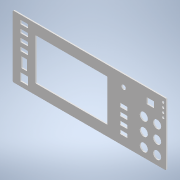
# Autodesk Inventor part: FrontPlate
Saved by Autodesk Inventor 2020.3 (Build 243373000, 373)
## iProperties
Created: 2021-02-28
Part Number: FrontPlate
Material: Generic
Document SubType Name: Modeling
Designer: vmiguel
Density: 1 g/cm^3
Appearance: Default
Author: vmiguel
Autodesk Inventor part; units mm, degrees
ref_plane "YZ Plane" through (0, 0, 0) normal (1, 0, 0) x (0, 1, 0)
ref_plane "XZ Plane" through (0, 0, 0) normal (0, 1, 0) x (-1, 0, 0)
ref_plane "XY Plane" through (0, 0, 0) normal (0, 0, 1) x (1, 0, 0)
sketch "Sketch1" plane through (0, 0, 0) normal (0, 0, 1) x (1, 0, 0)
  line L0 (-103.5, 42) -> (103.5, 42)
  line L1 (103.5, 42) -> (103.5, -42)
  line L2 (103.5, -42) -> (-103.5, -42)
  line L3 (-103.5, -42) -> (-103.5, 42)
  line L4 (-103.5, 42) -> (103.5, -42) construction
  line L5 (103.5, 42) -> (-103.5, -42) construction
  line L6 (-72.9, 28.2) -> (24.32, 28.2)
  line L7 (24.32, 28.2) -> (24.32, -28.2)
  line L8 (24.32, -28.2) -> (-72.9, -28.2)
  line L9 (-72.9, -28.2) -> (-72.9, 28.2)
  line L10 (-72.9, 28.2) -> (24.32, -28.2) construction
  line L11 (24.32, 28.2) -> (-72.9, -28.2) construction
  line L12 (-93.5, -25.4) -> (-82.9, -25.4)
  line L13 (-82.9, -25.4) -> (-82.9, -36)
  line L14 (-82.9, -36) -> (-93.5, -36)
  line L15 (-93.5, -36) -> (-93.5, -25.4)
  line L16 (-93.5, -25.4) -> (-82.9, -36) construction
  line L17 (-82.9, -25.4) -> (-93.5, -36) construction
  circle A0 centre (73.5, 6) radius 5.5
  circle A1 centre (91.5, 6) radius 5.5
  circle A2 centre (73.5, -12) radius 5.5
  circle A3 centre (91.5, -12) radius 5.5
  circle A4 centre (73.5, -30) radius 5.5
  circle A5 centre (91.5, -30) radius 5.5
  line L18 (-71.81, 26.93) -> (23.23, 26.93) construction
  line L19 (23.23, 26.93) -> (23.23, -26.93) construction
  line L20 (23.23, -26.93) -> (-71.81, -26.93) construction
  line L21 (-71.81, -26.93) -> (-71.81, 26.93) construction
  line L22 (-71.81, 26.93) -> (23.23, -26.93) construction
  line L23 (23.23, 26.93) -> (-71.81, -26.93) construction
  line L24 (-77, 32.18) -> (28.42, 32.18) construction
  line L25 (28.42, 32.18) -> (28.42, -34.89) construction
  line L26 (28.42, -34.89) -> (-77, -34.89) construction
  line L27 (-77, -34.89) -> (-77, 32.18) construction
  line L28 (-77, 32.18) -> (28.42, -34.89) construction
  line L29 (28.42, 32.18) -> (-77, -34.89) construction
  line L30 (-91.95, -19.9) -> (-84.45, -19.9)
  line L31 (-84.45, -19.9) -> (-84.45, -6)
  line L32 (-84.45, -6) -> (-91.95, -6)
  line L33 (-91.95, -6) -> (-91.95, -19.9)
  line L34 (-91.95, -19.9) -> (-84.45, -6) construction
  line L35 (-84.45, -19.9) -> (-91.95, -6) construction
  line L36 (-93.2, 4.5) -> (-83.2, 4.5)
  line L37 (-83.2, 4.5) -> (-83.2, -0.5)
  line L38 (-83.2, -0.5) -> (-93.2, -0.5)
  line L39 (-93.2, -0.5) -> (-93.2, 4.5)
  line L40 (-93.2, 4.5) -> (-83.2, -0.5) construction
  line L41 (-83.2, 4.5) -> (-93.2, -0.5) construction
  line L42 (-93.2, 15) -> (-83.2, 15)
  line L43 (-83.2, 15) -> (-83.2, 10)
  line L44 (-83.2, 10) -> (-93.2, 10)
  line L45 (-93.2, 10) -> (-93.2, 15)
  line L46 (-93.2, 15) -> (-83.2, 10) construction
  line L47 (-83.2, 15) -> (-93.2, 10) construction
  line L48 (-83.2, 20.5) -> (-93.2, 20.5)
  line L49 (-93.2, 20.5) -> (-93.2, 25.5)
  line L50 (-93.2, 25.5) -> (-83.2, 25.5)
  line L51 (-83.2, 25.5) -> (-83.2, 20.5)
  line L52 (-83.2, 20.5) -> (-93.2, 25.5) construction
  line L53 (-93.2, 20.5) -> (-83.2, 25.5) construction
  line L54 (-83.2, 36) -> (-93.2, 36)
  line L55 (-93.2, 36) -> (-93.2, 31)
  line L56 (-93.2, 31) -> (-83.2, 31)
  line L57 (-83.2, 31) -> (-83.2, 36)
  line L58 (-83.2, 36) -> (-93.2, 31) construction
  line L59 (-93.2, 36) -> (-83.2, 31) construction
  circle A6 centre (46.16, 26.75) radius 11 construction
  line L60 (68, 6) -> (68, -30) construction
  line L61 (24.32, -22.183) -> (68, -22.183) construction
  line L62 (73.5, 11.5) -> (91.5, 11.5) construction
  line L63 (82.5, 11.5) -> (82.5, 42) construction
  line L64 (77.5, 30.75) -> (87.5, 30.75)
  line L65 (87.5, 30.75) -> (87.5, 22.75)
  line L66 (87.5, 22.75) -> (77.5, 22.75)
  line L67 (77.5, 22.75) -> (77.5, 30.75)
  line L68 (77.5, 30.75) -> (87.5, 22.75) construction
  line L69 (87.5, 30.75) -> (77.5, 22.75) construction
  circle A7 centre (99.5, 35.75) radius 1.6
  circle A8 centre (99.5, 29.75) radius 1.6
  circle A9 centre (99.5, 23.75) radius 1.6
  circle A10 centre (99.5, 17.75) radius 1.6
  line L70 (99.5, 29.75) -> (99.5, 23.75) construction
  line L71 (41.16, -25.25) -> (51.16, -25.25)
  line L72 (51.16, -25.25) -> (51.16, -30.25)
  line L73 (51.16, -30.25) -> (41.16, -30.25)
  line L74 (41.16, -30.25) -> (41.16, -25.25)
  line L75 (41.16, -25.25) -> (51.16, -30.25) construction
  line L76 (51.16, -25.25) -> (41.16, -30.25) construction
  line L77 (41.16, -14.75) -> (51.16, -14.75)
  line L78 (51.16, -14.75) -> (51.16, -19.75)
  line L79 (51.16, -19.75) -> (41.16, -19.75)
  line L80 (41.16, -19.75) -> (41.16, -14.75)
  line L81 (41.16, -14.75) -> (51.16, -19.75) construction
  line L82 (51.16, -14.75) -> (41.16, -19.75) construction
  line L83 (51.16, -9.25) -> (41.16, -9.25)
  line L84 (41.16, -9.25) -> (41.16, -4.25)
  line L85 (41.16, -4.25) -> (51.16, -4.25)
  line L86 (51.16, -4.25) -> (51.16, -9.25)
  line L87 (51.16, -9.25) -> (41.16, -4.25) construction
  line L88 (41.16, -9.25) -> (51.16, -4.25) construction
  line L89 (51.16, 6.25) -> (41.16, 6.25)
  line L90 (41.16, 6.25) -> (41.16, 1.25)
  line L91 (41.16, 1.25) -> (51.16, 1.25)
  line L92 (51.16, 1.25) -> (51.16, 6.25)
  line L93 (51.16, 6.25) -> (41.16, 1.25) construction
  line L94 (41.16, 6.25) -> (51.16, 1.25) construction
  line L95 (46.16, -9.25) -> (46.16, -14.75) construction
  circle A11 centre (46.16, 26.75) radius 3
  point P0 (0, 0)
  point P1 (-24.29, 0)
  point P2 (0, 0)
  point P3 (-24.29, 0)
  point P4 (-88.2, -30.7)
  point P5 (-24.29, -1.355)
  point P6 (-88.2, -12.95)
  point P7 (-88.2, 2)
  point P8 (-88.2, 12.5)
  point P9 (-88.2, 23)
  point P10 (-88.2, 33.5)
  point P11 (-88.2, -12.95)
  point P12 (-88.2, -30.7)
  point P13 (-88.2, -12.95)
  point P14 (-88.2, 2)
  point P15 (-88.2, 2)
  point P16 (-88.2, 12.5)
  point P17 (-88.2, 12.5)
  point P18 (-88.2, 23)
  point P19 (-88.2, 23)
  point P20 (-88.2, 33.5)
  point P21 (46.16, -22.183)
  point P22 (82.5, 26.75)
  point P23 (87.5, 26.75)
  point P24 (99.5, 26.75)
  point P25 (46.16, -27.75)
  point P26 (46.16, -17.25)
  point P27 (46.16, -6.75)
  point P28 (46.16, 3.75)
  point P29 (46.16, -27.75)
  point P30 (46.16, -27.75)
  point P31 (46.16, -17.25)
  point P32 (46.16, -17.25)
  point P33 (46.16, -6.75)
  point P34 (46.16, -6.75)
  point P35 (46.16, 3.75)
  point P36 (46.16, 3.75)
  point P37 (46.16, -12)
  dimension "d11" = 11
  dimension "d0" = 207
  dimension "d1" = 84
  dimension "d4" = 56.4
  dimension "d5" = 97.22
  dimension "d6" = 10.6
  dimension "d7" = 10
  dimension "d8" = 6
  dimension "d9" = 18
  dimension "d10" = 18
  dimension "d12" = 18
  dimension "d13" = 95.04
  dimension "d14" = 53.86
  dimension "d15" = 5.19
  dimension "d16" = 3.98
  dimension "d17" = 67.07
  dimension "d18" = 105.42
  dimension "d21" = 10
  dimension "d22" = 12
  dimension "d23" = 12
  dimension "d24" = 13.9
  dimension "d25" = 7.5
  dimension "d26" = 5.5
  dimension "d27" = 5
  dimension "d28" = 5.5
  dimension "d29" = 5.5
  dimension "d30" = 5.5
  dimension "d31" = 5.5
  dimension "d32" = 10
  dimension "d33" = 6
  dimension "d34" = 22
  dimension "d35" = 10
  dimension "d36" = 8
  dimension "d37" = 3.2
  dimension "d38" = 3.2
  dimension "d39" = 3.2
  dimension "d40" = 3.2
  dimension "d41" = 6
  dimension "d42" = 6
  dimension "d43" = 6
  dimension "d44" = 4
  dimension "d45" = 5
  dimension "d46" = 5.5
  dimension "d47" = 5.5
  dimension "d48" = 5.5
  dimension "d49" = 10
  dimension "d52" = 6
  constraints: 192 end point, 58 midpoint, 30 parallel, 18 vertical alignment, 17 perpendicular, 16 horizontal, 10 centre point, 9 equal length, 8 horizontal alignment, 7 point on line, 2 equal radius, 2 point on circle, 2 tangent, 2 vertical, 1 coincident, 7 other
  measures "d0" distance of L1.end L2.end
  measures "d1" distance of L0.end L1.end
  measures "d4" distance of L6.end L7.end
  measures "d5" distance of L6.start L6.end
  measures "d6" distance of L12.start L12.end
  measures "d7" distance between parallel lines of L3 L15
  measures "d8" distance between parallel lines of L2 L14
  measures "d9" distance of point (91.5, 6) A0.centre
  measures "d10" distance of A0.centre A2.centre
  measures "d12" distance of point (73.5, -30) A2.centre
  measures "d13" distance of L19.end L20.end
  measures "d14" distance of L18.end L19.end
  measures "d15" distance between parallel lines of L27 L21
  measures "d16" distance between parallel lines of L6 L24
  measures "d17" distance of L26.end L24.start
  measures "d18" distance of L24.start L24.end
  measures "d21" distance between parallel lines of L9 L13
  measures "d22" distance from line of L1 point (91.5, 6)
  measures "d23" distance from line of A5.centre L2
  measures "d24" distance of L32.end L30.start
  measures "d25" distance of L31.end L32.end
  measures "d26" distance between parallel lines of L12 L30
  measures "d27" distance of L38.end L36.start
  measures "d28" distance between parallel lines of L32 L38
  measures "d29" distance between parallel lines of L44 L36
  measures "d30" distance between parallel lines of L42 L48
  measures "d31" distance between parallel lines of L50 L56
  measures "d32" distance of L54.start L54.end
  measures "d33" distance between parallel lines of L54 L0
  measures "d34" diameter of A6
  measures "d35" distance of L65.end L66.end
  measures "d36" distance of L64.end L65.end
  measures "d37" diameter of A7
  measures "d38" diameter of A8
  measures "d39" diameter of A9
  measures "d40" diameter of A10
  measures "d41" distance of L70.end L70.start
  measures "d42" distance of A7.centre L70.start
  measures "d43" distance of L70.end A10.centre
  measures "d44" distance from line of L1 A7.centre
  measures "d45" distance of L73.end L71.start
  measures "d46" distance between parallel lines of L79 L71
  measures "d47" distance between parallel lines of L77 L83
  measures "d48" distance between parallel lines of L85 L91
  measures "d49" distance of L89.start L90.start
  measures "d52" diameter of A11
extrude "Extrusion2" add sketch "Sketch1" along normal blind 1.6
fillet "Fillet1" radius 1 4 edges at (-103.5, 42, 0.8) (103.5, 42, 0.8) (103.5, -42, 0.8) (-103.5, -42, 0.8)
fillet "Fillet2" radius 0.75 4 edges at (-72.9, 28.2, 0.8) (24.32, 28.2, 0.8) (24.32, -28.2, 0.8) (-72.9, -28.2, 0.8)
fillet "Fillet3" radius 0.5 44 edges at (77.5, 30.75, 0.8) (87.5, 30.75, 0.8) (87.5, 22.75, 0.8) (77.5, 22.75, 0.8) (41.16, 6.25, 0.8) (51.16, 6.25, 0.8) (51.16, 1.25, 0.8) (41.16, 1.25, 0.8) (41.16, -4.25, 0.8) (51.16, -4.25, 0.8) (51.16, -9.25, 0.8) (41.16, -9.25, 0.8) (51.16, -14.75, 0.8) (51.16, -19.75, 0.8) (41.16, -14.75, 0.8) (41.16, -19.75, 0.8) (41.16, -30.25, 0.8) (41.16, -25.25, 0.8) (51.16, -25.25, 0.8) (51.16, -30.25, 0.8) (-93.5, -25.4, 0.8) (-93.5, -36, 0.8) (-82.9, -36, 0.8) (-82.9, -25.4, 0.8) (-84.45, -19.9, 0.8) (-91.95, -19.9, 0.8) (-91.95, -6, 0.8) (-84.45, -6, 0.8) (-83.2, -0.5, 0.8) (-93.2, -0.5, 0.8) (-93.2, 4.5, 0.8) (-83.2, 4.5, 0.8) (-83.2, 10, 0.8) (-83.2, 15, 0.8) (-93.2, 15, 0.8) (-93.2, 10, 0.8) (-93.2, 20.5, 0.8) (-83.2, 20.5, 0.8) (-83.2, 25.5, 0.8) (-93.2, 25.5, 0.8) (-83.2, 31, 0.8) (-83.2, 36, 0.8) (-93.2, 36, 0.8) (-93.2, 31, 0.8)
equation "\"d12\" = d10"
equation "\"d21\" = d7"
equation "\"d28\" = d26"
equation "\"d29\" = d28"
equation "\"d30\" = d29"
equation "\"d31\" = d29"
equation "\"d42\" = d41"
equation "\"d43\" = d41"
equation "\"d46\" = d50"
equation "\"d47\" = d46"
equation "\"d48\" = d46"
equation "\"d50\" = d51"
equation "\"d51\" = 5.5"
body "Solid2"
